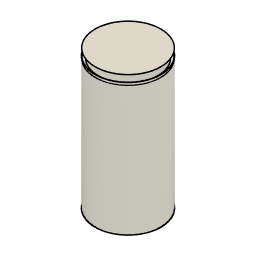
schibler-mathilde-2_carandache (Autodesk Fusion 360 design; units mm, degrees)
Autodesk Fusion 360 part; units mm, degrees
note: some values were not read from the file. Set by a fixed rule: which face or edge a step refers to.
sketch "Esquisse1" plane through (0, 0, 0) normal (0, 1, 0) x (1, 0, 0)
  circle A0 centre (0, 0) radius 250
  dimension "d1" = 500
  constraint coincident A0.centre origin
  measures "d1" diameter of A0
extrude "Extrusion1" add sketch "Esquisse1" along normal blind 1000 makes body 1
shell "Coque1" thickness 3 removed faces 1 at (36.3167, 1000, -54.8247) on bodies 1
shell "Coque2" thickness 3 removed faces 2 at (36.3167, 0, -54.8247) at (45.1812, 3, -17.7323) on bodies 1
sketch "Esquisse2" plane through (0, 0, 0) normal (0, 1, 0) x (1, 0, 0)
  circle A0 centre (0, 0) radius 247
  dimension "d6" = 494
  constraint coincident A0.centre origin
  measures "d6" diameter of A0
extrude "Extrusion2" add sketch "Esquisse2" along normal blind 3 separate body makes body 2
shell "Coque3" thickness 20 removed faces 2 at (-69.684, 3, 24.2682) at (-69.684, 0, 24.2682) on bodies 2
sketch "Esquisse3" plane through (0, 0, 0) normal (0, 1, 0) x (1, 0, 0)
  circle A0 centre (0, 0) radius 227
  dimension "d10" = 454
  constraint coincident A0.centre origin
  measures "d10" diameter of A0
extrude "Extrusion3" add sketch "Esquisse3" along normal blind 3 separate body makes body 3
copy_body "Copier/Coller des corps1" bodies 2 makes body 4
move_body "Déplacer1" bodies 4 to x (1, 0, 0) y (0, 1, 0) z (0, 0, 1) at (0, 0, 0)
move_body "Déplacer2" bodies 4 to x (1, 0, 0) y (0, 1, 0) z (0, 0, 1) at (0, 980, 0)
sketch "Esquisse6" plane through (0, 0, 0) normal (0, 1, 0) x (1, 0, 0)
  circle A0 centre (0, 0) radius 248
  dimension "d26" = 496
  constraint coincident A0.centre origin
  measures "d26" diameter of A0
extrude "Extrusion5" add sketch "Esquisse6" along normal blind 1 separate body makes body 5
move_body "Déplacer3" bodies 5 to x (1, 0, 0) y (0, 1, 0) z (0, 0, 1) at (0, 1050, 0)
sketch "Esquisse5" plane through (0, 10, 0) normal (0, 1, 0) x (-1, 0, 0)
  circle A0 centre (0, 0) radius 227
  circle A1 centre (0, 0) radius 247
  dimension "d25" = 494
  constraint concentric A0 A1
  measures "d25" diameter of A1
